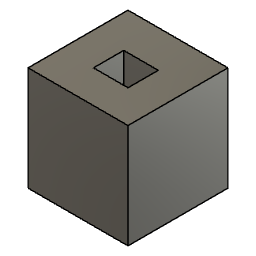
Imaging System Housing - Hikvision MV-CA013-20GM (Autodesk Fusion 360 design; units mm, degrees)
Autodesk Fusion 360 part; units mm, degrees
sketch "Sketch2" plane through (0, 0, 0) normal (0, 1, 0) x (1, 0, 0)
  line L0 (0, 0) -> (64.5, 0)
  line L1 (64.5, 0) -> (64.5, -35.5)
  line L2 (64.5, -35.5) -> (0, -35.5)
  line L3 (0, -35.5) -> (0, 0)
  dimension "d5" = 64.5
  dimension "d6" = 35.5
  constraint horizontal L0
  constraint vertical L1
  constraint horizontal L2
  constraint vertical L3
  constraint coincident L0.start L3.end
  measures "d5" distance of L0.start L0.end
  measures "d6" distance of L0.start L2.end
extrude "Extrude2" add sketch "Sketch2" along normal blind 100 makes body 1
sketch "Sketch3" plane through (0, 0, 0) normal (-1, 0, 0) x (0, 0, 1)
  line L0 (0, 0) -> (35.5, 0)
  line L1 (35.5, 0) -> (35.5, 100)
  line L2 (35.5, 100) -> (0, 100)
  line L3 (0, 100) -> (0, 0)
  line L4 (0, 100) -> (64.5, 100)
  line L5 (64.5, 100) -> (64.5, 0)
  line L6 (64.5, 0) -> (0, 0)
  line L7 (0, 0) -> (0, 100)
  dimension "d9" = 64.5
  dimension "d10" = 100
  constraint horizontal L4
  constraint vertical L5
  constraint horizontal L6
  constraint vertical L7
  constraint coincident L2.end L3.start
  measures "d9" distance of L2.end L4.end
  measures "d10" distance of L2.end L0.start
extrude "Extrude3" add sketch "Sketch3" along normal blind 31.4 separate body contours L1 L4 L5 L6 makes body 2
extrude "Extrude4" add 1 faces at (0, 66.6667, 23.6667) along direction (-1, 0, 0) blind 31.4 on bodies 1 bodies 1 2
sketch "Sketch4" plane through (0, 0, 64.5) normal (0, 0, 1) x (1, 0, 0)
  line L0 (0, 0) -> (0, 100)
  line L1 (0, 100) -> (-31.4, 100)
  line L2 (-31.4, 100) -> (-31.4, 0)
  line L3 (-31.4, 0) -> (0, 0)
  line L4 (-31.4, 100) -> (33.1, 100)
  line L5 (33.1, 100) -> (33.1, 0)
  line L6 (33.1, 0) -> (-31.4, 0)
  line L7 (-31.4, 0) -> (-31.4, 100)
  dimension "d15" = 64.5
  dimension "d16" = 100
  constraint horizontal L4
  constraint vertical L5
  constraint horizontal L6
  constraint vertical L7
  constraint coincident L1.end L2.start
  measures "d15" distance of L1.end L4.end
  measures "d16" distance of L1.end L2.end
extrude "Extrude5" add sketch "Sketch4" along normal blind 31.4 bodies 1
sketch "Sketch5" plane through (33.1, 0, 0) normal (1, 0, 0) x (0, 0, -1)
  line L0 (-64.5, 0) -> (-64.5, 100)
  line L1 (-64.5, 100) -> (-95.9, 100)
  line L2 (-95.9, 100) -> (-95.9, 0)
  line L3 (-95.9, 0) -> (-64.5, 0)
  line L4 (-95.9, 100) -> (-31.4, 100)
  line L5 (-31.4, 100) -> (-31.4, 0)
  line L6 (-31.4, 0) -> (-95.9, 0)
  line L7 (-95.9, 0) -> (-95.9, 100)
  dimension "d19" = 64.5
  dimension "d20" = 100
  constraint horizontal L4
  constraint vertical L5
  constraint horizontal L6
  constraint vertical L7
  constraint coincident L1.end L2.start
  measures "d19" distance of L1.end L4.end
  measures "d20" distance of L1.end L2.end
extrude "Extrude6" add sketch "Sketch5" along normal blind 31.4 bodies 1
